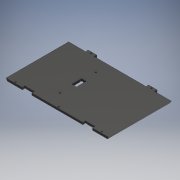
# Autodesk Inventor part: BA14
Saved by Autodesk Inventor 2017 (Build 210142000, 142)
## iProperties
Created: 2019-05-29
Part Number: BA14
Material: Wood (Cherry)
Document SubType Name: Modeling
Designer: Dell
Density: 0.63 g/cm^3
Appearance: Smooth - Black
Mass: 220.188 g
Surface Area: 1174.42 cm^2
Volume: 349.504 cm^3
Author: Dell
Autodesk Inventor part; units mm, degrees
ref_plane "YZ Plane" through (0, 0, 0) normal (1, 0, 0) x (0, 1, 0)
sketch "Sketch1" plane through (0, 0, 0) normal (0, 0, 1) x (1, 0, 0)
  line L0 (0, 0) -> (303.5647, 0)
  line L1 (303.5647, 0) -> (303.5647, 184.15)
  line L2 (303.5647, 184.15) -> (0, 184.15)
  line L3 (0, 184.15) -> (0, 0)
  dimension "d0" = 303.5647
  dimension "d1" = 184.15
  constraints: 8 end point, 2 parallel, 1 horizontal, 1 perpendicular
  measures "d0" distance of L0.start L0.end
  measures "d1" distance of L2.end L0.start
extrude "Extrusion1" add sketch "Sketch1" along normal blind 6.35
sketch "Sketch2" plane through (0, 184.15, 0) normal (0, 1, 0) x (1, 0, 0)
  line L0 (0, -6.35) -> (303.5647, -6.35) projected
  line L1 (0, -6.35) -> (3.6662, 0)
  line L2 (3.6662, 0) -> (0, 0)
  line L3 (0, 0) -> (0, -6.35)
  line L4 (0, 0) -> (303.5647, 0) projected
  line L5 (303.5647, 0) -> (303.5647, -6.35) projected
  line L6 (299.8985, 0) -> (303.5647, -6.35)
  line L7 (303.5647, -6.35) -> (303.5647, 0)
  line L8 (303.5647, 0) -> (299.8985, 0)
  dimension "d4" = 30
  dimension "d5" = 30
  constraints: 12 end point, 2 perpendicular, 1 collinear, 1 parallel, 1 point on line
  measures "d4" angle of L5 L6
  measures "d5" angle of L3 L1
extrude "Extrusion2" cut sketch "Sketch2" against normal through all contours L3 L2 L1 | L6 L4 L5
ref_plane "Work Plane1" through (3.6662, 92.075, 0) normal (0, -1, 0) x (1, 0, 0)
sketch "Sketch4" plane through (3.6662, 92.075, 0) normal (0, -1, 0) x (1, 0, 0)
  line L0 (0, 0) -> (296.2324, 0) projected
  line L1 (118.4324, 0) -> (129.4309, 6.35) construction
  line L2 (129.4309, 6.35) -> (116.7309, 6.35) construction
  line L3 (-3.6662, 6.35) -> (299.8985, 6.35) projected
  line L4 (118.4324, 0) -> (111.1, 0)
  line L5 (118.0728, 4.0257) -> (111.1, 0) construction
  line L6 (-3.6662, 6.35) -> (0, 0) projected
  line L7 (118.4324, 0) -> (122.0985, 6.35)
  line L8 (111.1, 0) -> (114.7662, 6.35)
  line L9 (122.0985, 6.35) -> (114.7662, 6.35)
  point P0 (-3.6662, 0)
  dimension "d13" = 88.9
  dimension "d14" = 30
  dimension "d15" = 60
  dimension "d16" = 6.35
  constraints: 14 end point, 5 point on line, 2 parallel
  measures "d13" distance from line of L0.end L1
  measures "d14" angle of L0 L1
  measures "d15" angle of L0 L7
  measures "d16" distance between parallel lines of L7 L8
extrude "Extrusion3" cut sketch "Sketch4" along normal blind 9.525 and the other way blind 15.875 contours L8 L3 L7 L0
sketch "Sketch5" plane through (0, 0, 6.35) normal (0, 0, 1) x (1, 0, 0)
  line L0 (3.6662, 0) -> (299.8985, 0) projected
  line L1 (50.1824, 0) -> (75.5824, 0)
  line L2 (75.5824, 0) -> (75.5824, 7.62)
  line L3 (75.5824, 7.62) -> (50.1824, 7.62)
  line L4 (50.1824, 7.62) -> (50.1824, 0)
  line L5 (227.9824, 0) -> (253.3824, 0)
  line L6 (253.3824, 0) -> (253.3824, 7.62)
  line L7 (253.3824, 7.62) -> (227.9824, 7.62)
  line L8 (227.9824, 7.62) -> (227.9824, 0)
  line L9 (75.5824, 7.62) -> (227.9824, 7.62) construction
  point P0 (0, 0)
  point P1 (151.7824, 7.62)
  point P2 (151.7824, 0)
  dimension "d19" = 25.4
  dimension "d20" = 7.62
  dimension "d21" = 25.4
  dimension "d22" = 7.62
  dimension "d23" = 152.4
  constraints: 18 end point, 4 parallel, 2 horizontal, 2 midpoint, 2 perpendicular, 2 point on line, 1 vertical alignment
  measures "d19" distance of L3.end L2.end
  measures "d20" distance of L2.end L1.end
  measures "d21" distance of L7.end L6.end
  measures "d22" distance of L6.end L5.end
  measures "d23" distance of L2.end L7.end
extrude "Extrusion4" cut sketch "Sketch5" against normal through all
sketch "Sketch6" plane through (0, 0, 6.35) normal (0, 0, 1) x (1, 0, 0)
  line L0 (299.8985, 184.15) -> (3.6662, 184.15) projected
  line L1 (50.1824, 184.15) -> (75.5824, 184.15)
  line L2 (75.5824, 184.15) -> (75.5824, 191.77)
  line L3 (75.5824, 191.77) -> (50.1824, 191.77)
  line L4 (50.1824, 191.77) -> (50.1824, 184.15)
  line L5 (50.1824, 7.62) -> (75.5824, 7.62) projected
  line L6 (227.9824, 184.15) -> (253.3824, 184.15)
  line L7 (253.3824, 184.15) -> (253.3824, 191.77)
  line L8 (253.3824, 191.77) -> (227.9824, 191.77)
  line L9 (227.9824, 191.77) -> (227.9824, 184.15)
  line L10 (227.9824, 7.62) -> (253.3824, 7.62) projected
  point P0 (0, 0)
  point P1 (62.8824, 191.77)
  point P2 (62.8824, 7.62)
  point P3 (240.6824, 191.77)
  point P4 (240.6824, 7.62)
  dimension "d26" = 25.4
  dimension "d27" = 7.62
  dimension "d28" = 25.4
  dimension "d29" = 7.62
  constraints: 16 end point, 4 midpoint, 4 parallel, 2 horizontal, 2 perpendicular, 2 point on line, 2 vertical alignment
  measures "d26" distance of L3.end L2.end
  measures "d27" distance of L2.end L1.end
  measures "d28" distance of L8.end L7.end
  measures "d29" distance of L7.end L6.end
extrude "Extrusion5" add sketch "Sketch6" against normal blind 6.35
ref_plane "Work Plane2" through (125.7647, 92.075, 6.35) normal (-0.5, 0, -0.8660254) x (0, -1, 0)
sketch "Sketch7" plane through (125.7647, 92.075, 6.35) normal (-0.5, 0, -0.8660254) x (0, -1, 0)
  line L0 (-15.875, 6.35) -> (-15.875, 0) projected
  line L1 (-15.875, 3.175) -> (-92.075, 3.175) construction
  line L2 (-92.075, -88.5231) -> (-92.075, 43.4592) projected
  line L3 (9.525, 0) -> (9.525, 6.35) projected
  line L4 (9.525, 3.175) -> (92.075, 3.175) construction
  line L5 (92.075, 43.4592) -> (92.075, -88.5231) projected
  circle A0 centre (-53.975, 3.175) radius 2.25
  circle A1 centre (50.8, 3.175) radius 2.25
  point P0 (92.075, 105.7404)
  dimension "d33" = 4.5
  dimension "d34" = 4.5
  constraints: 4 end point, 4 midpoint, 3 point on line, 2 centre point, 1 horizontal
  measures "d33" diameter of A0
  measures "d34" diameter of A1
extrude "Extrusion6" cut sketch "Sketch7" along normal through all
sketch "Sketch8" plane through (0, 0, 6.35) normal (0, 0, 1) x (1, 0, 0)
  circle A0 centre (62.8824, 187.96) radius 2.25
  circle A1 centre (240.6824, 187.96) radius 2.25
  circle A2 centre (278.4735, 3.81) radius 2.25
  circle A3 centre (151.7824, 3.81) radius 2.25
  circle A4 centre (25.0912, 3.81) radius 2.25
  line L0 (0, 0) -> (50.1824, 0) projected
  line L1 (75.5824, 0) -> (227.9824, 0) projected
  line L2 (253.3824, 0) -> (303.5647, 0) projected
  line L3 (50.1824, 0) -> (50.1824, 7.62) projected
  line L4 (253.3824, 184.15) -> (253.3824, 191.77) projected
  line L5 (75.5824, 191.77) -> (50.1824, 191.77) projected
  line L6 (253.3824, 191.77) -> (227.9824, 191.77) projected
  point P0 (25.0912, 0)
  point P1 (151.7824, 0)
  point P2 (278.4735, 0)
  point P3 (50.1824, 3.81)
  point P4 (253.3824, 187.96)
  point P5 (62.8824, 191.77)
  point P6 (240.6824, 191.77)
  dimension "d37" = 4.5
  dimension "d38" = 4.5
  dimension "d39" = 4.5
  dimension "d40" = 4.5
  dimension "d41" = 4.5
  constraints: 7 midpoint, 5 centre point, 5 horizontal alignment, 5 vertical alignment
  measures "d37" diameter of A0
  measures "d38" diameter of A1
  measures "d39" diameter of A2
  measures "d40" diameter of A3
  measures "d41" diameter of A4
extrude "Extrusion7" cut sketch "Sketch8" against normal through all
sketch "Sketch9" plane through (0, 0, 0) normal (0, 0, -1) x (-1, 0, 0)
  ellipse E0 centre (-118.4324, 41.275) end of major axis (-121.0304, 41.275) minor radius 2.25 projected
  line L0 (-114.7662, 107.95) -> (-114.7662, 82.55) projected
  line L1 (-114.7662, 107.95) -> (-118.4324, 107.95) projected
  line L2 (-118.4324, 82.55) -> (-118.4324, 107.95) projected
  line L3 (-118.4324, 82.55) -> (-114.7662, 82.55) projected
  ellipse E1 centre (-118.4324, 146.05) end of major axis (-121.0304, 146.05) minor radius 2.25 projected
  point P0 (0, 0)
  constraints: 2 other
extrude "Extrusion8" cut sketch "Sketch9" along normal through all both and the other way through all
sketch "Sketch10" plane through (0, 0, 6.35) normal (0, 0, 1) x (1, 0, 0)
  ellipse E0 centre (118.4324, 146.05) end of major axis (115.8343, 146.05) minor radius 2.25 (118.4324, 143.8) -> (120.2654, 144.4555) ccw projected
  ellipse E1 centre (122.0985, 146.05) end of major axis (124.6966, 146.05) minor radius 2.25 (120.2654, 144.4555) -> (120.2654, 147.6445) ccw projected
  ellipse E2 centre (118.4324, 146.05) end of major axis (115.8343, 146.05) minor radius 2.25 (120.2654, 147.6445) -> (118.4324, 148.3) ccw projected
  ellipse E3 centre (118.4324, 146.05) end of major axis (121.0304, 146.05) minor radius 2.25 (118.4324, 143.8) -> (118.4324, 148.3) ccw projected
  ellipse E4 centre (118.4324, 41.275) end of major axis (115.8343, 41.275) minor radius 2.25 (118.4324, 39.025) -> (120.2654, 39.6805) ccw projected
  ellipse E5 centre (122.0985, 41.275) end of major axis (124.6966, 41.275) minor radius 2.25 (120.2654, 39.6805) -> (120.2654, 42.8695) ccw projected
  ellipse E6 centre (118.4324, 41.275) end of major axis (115.8343, 41.275) minor radius 2.25 (120.2654, 42.8695) -> (118.4324, 43.525) ccw projected
  ellipse E7 centre (118.4324, 41.275) end of major axis (121.0304, 41.275) minor radius 2.25 (118.4324, 39.025) -> (118.4324, 43.525) ccw projected
  line L0 (125.7647, 107.95) -> (125.7647, 82.55) projected
  line L1 (125.7647, 107.95) -> (122.0985, 107.95) projected
  line L2 (122.0985, 82.55) -> (122.0985, 107.95) projected
  line L3 (122.0985, 82.55) -> (125.7647, 82.55) projected
  point P0 (0, 0)
  constraints: 8 other
extrude "Extrusion9" cut sketch "Sketch10" against normal through all contours L0 L3 L2 L1
sketch "Sketch11" plane through (0, 0, 6.35) normal (0, 0, 1) x (1, 0, 0)
  ellipse E0 centre (118.4324, 146.05) end of major axis (115.8343, 146.05) minor radius 2.25 (120.2654, 147.6445) -> (120.2654, 144.4555) ccw projected
  ellipse E1 centre (118.4324, 41.275) end of major axis (115.8343, 41.275) minor radius 2.25 (120.2654, 42.8695) -> (120.2654, 39.6805) ccw projected
  circle A0 centre (118.4324, 41.275) radius 2.25
  circle A1 centre (118.4324, 146.05) radius 2.25
  circle A2 centre (118.4324, 146.05) radius 7.5
  circle A3 centre (118.4324, 41.275) radius 7.5
  point P0 (0, 0)
  dimension "d48" = 4.5
  dimension "d49" = 4.5
  dimension "d50" = 15
  dimension "d51" = 15
  constraints: 4 centre point, 4 coincident, 2 other
  measures "d48" diameter of A0
  measures "d49" diameter of A1
  measures "d50" diameter of A2
  measures "d51" diameter of A3
extrude "Extrusion10" add sketch "Sketch11" against normal up to surface (6.35 mm away) from surface at 0 contours A1 E0 | A0 E1 | A2 | A3
sketch "Sketch12" plane through (0, 0, 6.35) normal (0, 0, 1) x (1, 0, 0)
  line L0 (3.6662, 0) -> (50.1824, 0) projected
  line L1 (48.9124, 0) -> (76.8524, 0)
  line L2 (76.8524, 0) -> (76.8524, 7.62)
  line L3 (76.8524, 7.62) -> (48.9124, 7.62)
  line L4 (48.9124, 7.62) -> (48.9124, 0)
  line L5 (75.5824, 0) -> (227.9824, 0) projected
  line L6 (226.7124, 0) -> (254.6524, 0)
  line L7 (254.6524, 0) -> (254.6524, 7.62)
  line L8 (254.6524, 7.62) -> (226.7124, 7.62)
  line L9 (226.7124, 7.62) -> (226.7124, 0)
  line L10 (50.1824, 7.62) -> (75.5824, 7.62) projected
  line L11 (227.9824, 7.62) -> (253.3824, 7.62) projected
  line L12 (50.1824, 0) -> (50.1824, 7.62) projected
  line L13 (227.9824, 0) -> (227.9824, 7.62) projected
  line L14 (114.7662, 107.95) -> (125.7647, 107.95) projected
  line L15 (114.7662, 82.55) -> (114.7662, 107.95) projected
  line L16 (125.7647, 82.55) -> (114.7662, 82.55) projected
  line L17 (125.7647, 107.95) -> (125.7647, 82.55) projected
  line L18 (113.4962, 109.22) -> (127.0347, 109.22)
  line L19 (127.0347, 109.22) -> (127.0347, 81.28)
  line L20 (127.0347, 81.28) -> (113.4962, 81.28)
  line L21 (113.4962, 81.28) -> (113.4962, 109.22)
  point P0 (0, 0)
  point P1 (62.8824, 7.62)
  point P2 (240.6824, 7.62)
  dimension "d54" = 1.27
  dimension "d55" = 1.27
  dimension "d56" = 1.27
  constraints: 24 end point, 4 midpoint, 4 parallel, 3 point on line, 2 horizontal, 2 perpendicular, 3 other
  measures "d54" distance between parallel lines of L4 L12
  measures "d55" distance between parallel lines of L13 L9
  measures "d56" distance between parallel lines of L15 L21
extrude "Extrusion11" cut sketch "Sketch12" against normal through all contours L4 L3 L12 L0 | L12 L3 L2 L1 | L9 L8 L13 L5 | L13 L8 L7 L6 | L14 L17 L16 L15 | L18 L19 L20 L21
sketch "Sketch13" plane through (0, 0, 6.35) normal (0, 0, 1) x (1, 0, 0)
  line L0 (254.6524, 7.62) -> (254.6524, 0) construction
  line L1 (254.6524, 0) -> (303.5647, 0) construction
  line L2 (303.5647, 0) -> (303.5647, 184.15) construction
  line L3 (303.5647, 184.15) -> (253.3824, 184.15) construction
  line L4 (253.3824, 184.15) -> (253.3824, 191.77) construction
  line L5 (253.3824, 191.77) -> (227.9824, 191.77) construction
  line L6 (227.9824, 191.77) -> (227.9824, 184.15) construction
  line L7 (227.9824, 184.15) -> (75.5824, 184.15) construction
  line L8 (75.5824, 184.15) -> (75.5824, 191.77) construction
  line L9 (75.5824, 191.77) -> (50.1824, 191.77) construction
  line L10 (50.1824, 191.77) -> (50.1824, 184.15) construction
  line L11 (50.1824, 184.15) -> (0, 184.15) construction
  line L12 (0, 184.15) -> (0, 0) construction
  line L13 (0, 0) -> (48.9124, 0) construction
  line L14 (48.9124, 0) -> (48.9124, 7.62) construction
  line L15 (48.9124, 7.62) -> (76.8524, 7.62) construction
  line L16 (76.8524, 7.62) -> (76.8524, 0) construction
  line L17 (76.8524, 0) -> (226.7124, 0) construction
  line L18 (226.7124, 0) -> (226.7124, 7.62) construction
  line L19 (226.7124, 7.62) -> (254.6524, 7.62) construction
  line L20 (113.4962, 81.28) -> (113.4962, 109.22) construction
  line L21 (113.4962, 109.22) -> (127.0347, 109.22) construction
  line L22 (127.0347, 109.22) -> (127.0347, 81.28) construction
  line L23 (127.0347, 81.28) -> (113.4962, 81.28) construction
  circle A0 centre (118.4324, 146.05) radius 2.25 construction
  circle A1 centre (118.4324, 41.275) radius 2.25 construction
  circle A2 centre (25.0912, 3.81) radius 2.25 construction
  circle A3 centre (278.4735, 3.81) radius 2.25 construction
  circle A4 centre (62.8824, 187.96) radius 2.25 construction
  circle A5 centre (240.6824, 187.96) radius 2.25 construction
  circle A6 centre (151.7824, 3.81) radius 2.25 construction
  line L24 (77.8274, 186.3951) -> (225.7373, 186.3951) construction
  line L25 (225.7373, 186.3951) -> (225.7373, 194.0151) construction
  line L26 (225.7373, 194.0151) -> (255.6274, 194.0151) construction
  line L27 (255.6274, 194.0151) -> (255.6274, 186.3951) construction
  line L28 (255.6274, 186.3951) -> (305.8098, 186.3951) construction
  line L29 (305.8098, 186.3951) -> (305.8098, -2.2451) construction
  line L30 (305.8098, -2.2451) -> (252.4073, -2.2451) construction
  line L31 (252.4073, -2.2451) -> (252.4073, 5.3749) construction
  line L32 (252.4073, 5.3749) -> (228.9574, 5.3749) construction
  line L33 (228.9574, 5.3749) -> (228.9574, -2.2451) construction
  line L34 (228.9574, -2.2451) -> (74.6073, -2.2451) construction
  line L35 (74.6073, -2.2451) -> (74.6073, 5.3749) construction
  line L36 (74.6073, 5.3749) -> (51.1574, 5.3749) construction
  line L37 (51.1574, 5.3749) -> (51.1574, -2.2451) construction
  line L38 (51.1574, -2.2451) -> (-2.2451, -2.2451) construction
  line L39 (-2.2451, -2.2451) -> (-2.2451, 186.3951) construction
  line L40 (-2.2451, 186.3951) -> (47.9373, 186.3951) construction
  line L41 (47.9373, 186.3951) -> (47.9373, 194.0151) construction
  line L42 (47.9373, 194.0151) -> (77.8274, 194.0151) construction
  line L43 (77.8274, 194.0151) -> (77.8274, 186.3951) construction
  circle A7 centre (47.9373, 186.3951) radius 3.175
  circle A8 centre (77.8274, 186.3951) radius 3.175
  circle A9 centre (225.7373, 186.3951) radius 3.175
  circle A10 centre (255.6274, 186.3951) radius 3.175
  circle A11 centre (252.4073, 5.3749) radius 3.175
  line L44 (226.7124, 7.62) -> (254.6524, 7.62) projected
  circle A12 centre (228.9574, 5.3749) radius 3.175
  line L45 (48.9124, 7.62) -> (76.8524, 7.62) projected
  circle A13 centre (74.6073, 5.3749) radius 3.175
  circle A14 centre (51.1574, 5.3749) radius 3.175
  line L46 (115.7412, 106.9749) -> (115.7412, 83.5251) construction
  line L47 (115.7412, 83.5251) -> (124.7896, 83.5251) construction
  line L48 (124.7896, 83.5251) -> (124.7896, 106.9749) construction
  line L49 (124.7896, 106.9749) -> (115.7412, 106.9749) construction
  line L50 (113.4962, 109.22) -> (113.4962, 81.28) projected
  circle A15 centre (115.7412, 106.9749) radius 3.175
  circle A16 centre (124.7896, 106.9749) radius 3.175
  line L51 (127.0347, 81.28) -> (127.0347, 109.22) projected
  circle A17 centre (124.7896, 83.5251) radius 3.175
  circle A18 centre (115.7412, 83.5251) radius 3.175
  dimension "d59" = 6.35
  dimension "d60" = 6.35
  constraints: 48 end point, 12 coincident, 58 other
extrude "Extrusion12" cut sketch "Sketch13" along normal through all both and the other way through all
sketch "Sketch14" plane through (80.0725, 184.15, 0) normal (0, 1, 0) x (1, 0, 0)
  line L0 (-76.4063, 0) -> (-80.0725, -6.35) projected
  line L1 (-80.0725, -6.35) -> (-79.3392, -6.35)
  line L2 (-80.0725, -6.35) -> (-31.1601, -6.35) construction
  line L3 (-79.3392, -6.35) -> (-75.6731, 0)
  line L4 (-76.4063, 0) -> (-31.1601, 0) construction
  line L5 (-75.6731, 0) -> (-76.4063, 0)
  line L6 (174.5799, -6.35) -> (223.4922, -6.35) construction
  line L7 (223.4922, -6.35) -> (222.759, -6.35)
  line L8 (222.759, -6.35) -> (219.0928, 0)
  line L9 (219.8261, 0) -> (177.8, 0) construction
  line L10 (219.0928, 0) -> (219.8261, 0)
  line L11 (223.4922, -6.35) -> (219.8261, 0) projected
  line L12 (219.8261, 0) -> (223.4922, -6.35)
  point P0 (-80.0725, 0)
  dimension "d63" = 0.635
  dimension "d64" = 0.635
  constraints: 14 end point, 3 parallel, 2 collinear, 2 point on line
  measures "d63" distance between parallel lines of L3 L0
  measures "d64" distance between parallel lines of L11 L8
extrude "Extrusion13" cut sketch "Sketch14" against normal through all
equation "\"d2\" = Panel_Thickness"
equation "\"d16\" = Panel_Thickness"
equation "\"d20\" = Panel_Thickness + Fit_Tolerance"
equation "\"d22\" = Panel_Thickness + Fit_Tolerance"
equation "\"d27\" = Panel_Thickness + Fit_Tolerance"
equation "\"d29\" = Panel_Thickness + Fit_Tolerance"
equation "\"d30\" = Panel_Thickness"
equation "\"d35\" = Panel_Thickness"
equation "\"d42\" = Panel_Thickness"
equation "\"d46\" = Panel_Thickness"
equation "\"d52\" = Panel_Thickness"
equation "\"d54\" = Fit_Tolerance"
equation "\"d55\" = Fit_Tolerance"
equation "\"d56\" = Fit_Tolerance"
equation "\"d57\" = Panel_Thickness"
equation "\"d59\" = Tool_Dia"
equation "\"d60\" = Tool_Dia"
equation "\"d63\" = 0.5 * Fit_Tolerance"
equation "\"d64\" = 0.5 * Fit_Tolerance"
equation "\"d65\" = Panel_Thickness"
equation "\"Panel_Thickness\" = 6.35"
equation "\"Fit_Tolerance\" = 1.27"
equation "\"Tool_Dia\" = 6.35"
body "Solid1"
